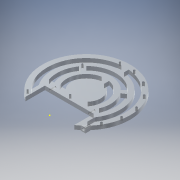
# Autodesk Inventor part: M02_R01 - Main Spherical Shaft
Saved by Autodesk Inventor 2016 (Build 200138000, 138)
## iProperties
Created: 2017-02-27
Part Number: M02_R01 - Main Spherical Shaft
Material: Glass
Document SubType Name: Modeling
Designer: Fernando
Stock Number: 0
Mass: 238.84 g
Surface Area: 460.743 cm^2
Volume: 109.56 cm^3
Density: 2.18 g/cm^3
Appearance: Clear
SurfaceArea_m2: .05
Author: Fernando
Autodesk Inventor part; units mm, degrees
ref_plane "YZ Plane" through (0, 0, 0) normal (1, 0, 0) x (0, 1, 0)
ref_plane "XZ Plane" through (0, 0, 0) normal (0, 1, 0) x (-1, 0, 0)
ref_plane "XY Plane" through (0, 0, 0) normal (0, 0, 1) x (1, 0, 0)
sketch "Sketch2" plane through (0, 0, 0) normal (0, 0, 1) x (1, 0, 0)
  line L0 (-50, 0) -> (50, 0) construction
  line L1 (50, 0) -> (50, 40)
  line L2 (50, 40) -> (-50, 40)
  line L3 (-50, 40) -> (-50, 0)
  arc A0 (50, 0) -> (-50, 0) centre (0, 74.8331) ccw
  line L4 (57.5, 19.2117) -> (57.5, 34.9113)
  line L5 (-57.5, 34.9113) -> (-57.5, 19.2117)
  line L6 (7.5, 154.4808) -> (7.5, 144.4302)
  line L7 (-7.5, 154.4808) -> (-7.5, 144.4302)
  line L8 (7.5, 144.4302) -> (-7.5, 154.4808) construction
  arc A1 (57.5, 34.9113) -> (7.5, 144.4302) centre (0, 74.8331) ccw
  arc A2 (-7.5, 144.4302) -> (-57.5, 34.9113) centre (0, 74.8331) ccw
  arc A3 (57.5, 19.2117) -> (7.5, 154.4808) centre (0, 74.8331) ccw
  arc A4 (-7.5, 154.4808) -> (-57.5, 19.2117) centre (0, 74.8331) ccw
  line L9 (56.6273, 55) -> (45.8982, 55)
  line L10 (-45.8982, 55) -> (-56.6273, 55)
  line L11 (42.4264, 117.2596) -> (35.3553, 110.1885)
  line L12 (-35.3553, 110.1885) -> (-42.4264, 117.2596)
  line L13 (49.1491, 109.2477) -> (40.9576, 103.512)
  line L14 (-49.1491, 109.2477) -> (-40.9576, 103.512)
  arc A5 (-40.9576, 103.512) -> (-45.8982, 55) centre (0, 74.8331) ccw
  arc A6 (-49.1491, 109.2477) -> (-56.6273, 55) centre (0, 74.8331) ccw
  arc A7 (45.8982, 55) -> (40.9576, 103.512) centre (0, 74.8331) ccw
  arc A8 (35.3553, 110.1885) -> (-35.3553, 110.1885) centre (0, 74.8331) ccw
  arc A9 (56.6273, 55) -> (49.1491, 109.2477) centre (0, 74.8331) ccw
  arc A10 (42.4264, 117.2596) -> (-42.4264, 117.2596) centre (0, 74.8331) ccw
  line L15 (7.5, 114.1237) -> (7.5, 103.8805)
  line L16 (-7.5, 103.8805) -> (-7.5, 114.1237)
  line L17 (34.7368, 55) -> (22.5088, 55)
  line L18 (-22.5088, 55) -> (-34.7368, 55)
  arc A11 (-7.5, 103.8805) -> (-22.5088, 55) centre (0, 74.8331) ccw
  arc A12 (22.5088, 55) -> (7.5, 103.8805) centre (0, 74.8331) ccw
  arc A13 (-7.5, 114.1237) -> (-34.7368, 55) centre (0, 74.8331) ccw
  arc A14 (34.7368, 55) -> (7.5, 114.1237) centre (0, 74.8331) ccw
  point P0 (0, 0)
  point P1 (0, 0)
  point P2 (0, 149.4555)
  dimension "d11" = 100
  dimension "d12" = 40
  dimension "d27" = 90
  dimension "d29" = 7.5
  dimension "d30" = 7.5
  dimension "d34" = 10
  dimension "d35" = 10
  dimension "d36" = 10
  dimension "d37" = 10
  dimension "d38" = 15
  dimension "d71" = 15
  dimension "d74" = 10
  dimension "d75" = 10
  dimension "d76" = 45
  dimension "d77" = 45
  dimension "d78" = 10
  dimension "d79" = 10
  dimension "d80" = 10
  dimension "d81" = 10
  constraints: 38 end point, 30 point on circle, 15 centre point, 7 coincident, 6 concentric, 5 collinear, 5 parallel, 4 point on line, 4 vertical, 3 horizontal, 2 midpoint, 1 perpendicular, 1 vertical alignment
  measures "d11" distance of L0.start L0.end
  measures "d12" distance of L0.end L1.end
  measures "d27" radius of A0
  measures "d29" distance between parallel lines of L1 L4
  measures "d30" distance between parallel lines of L3 L5
  measures "d34" radial gap between concentric circles of A0 A3
  measures "d35" radial gap between concentric circles of A3 A1
  measures "d36" radial gap between concentric circles of A4 A2
  measures "d37" radial gap between concentric circles of A0 A4
  measures "d38" distance between parallel lines of L7 L6
  measures "d71" distance between parallel lines of L2 L10
  measures "d74" angle of L13 L11
  measures "d75" angle of L14 L12
  measures "d76" angle of L2 L11
  measures "d77" angle of L2 L12
  measures "d78" radial gap between concentric circles of A1 A10
  measures "d79" radial gap between concentric circles of A8 A10
  measures "d80" radial gap between concentric circles of A7 A14
  measures "d81" radial gap between concentric circles of A12 A14
extrude "Extrusion2" add sketch "Sketch2" along normal mid plane 8
sketch "Sketch6" plane through (0, 0, 0) normal (0, 0, 1) x (1, 0, 0)
  arc A0 (50, 0) -> (-50, 0) centre (0, 74.8331) ccw projected
  line L0 (57.5, 5.5962) -> (67.5, 5.5962)
  line L1 (67.5, 5.5962) -> (67.5, 15.3037)
  point P0 (0, 0)
  point P1 (57.5, 19.2117)
  dimension "d48" = 10
  constraints: 4 end point, 2 point on circle, 1 horizontal, 1 perpendicular, 1 vertical alignment
  measures "d48" distance of L0.start L0.end
extrude "Extrusion4" add sketch "Sketch6" along normal mid plane 10
sketch "Sketch8" plane through (0, 0, 0) normal (0, 0, 1) x (1, 0, 0)
  arc A0 (50, 0) -> (-50, 0) centre (0, 74.8331) ccw construction
  line L0 (2, 165.8331) -> (0, 163.8331)
  line L1 (0, 163.8331) -> (-2, 165.8331)
  line L2 (-2, 165.8331) -> (2, 165.8331)
  line L3 (0, 165.8331) -> (0, 164.8331) construction
  point P0 (0, 0)
  point P1 (67.5, 15.3037)
  dimension "d67" = 1
  dimension "d68" = 2
  constraints: 8 end point, 2 perpendicular, 1 horizontal, 1 midpoint, 1 point on circle, 1 vertical, 1 vertical alignment
  measures "d67" distance of L3.start L3.end
  measures "d68" distance from line of L2 L0.end
extrude "Extrusion5" cut sketch "Sketch8" along normal mid plane 10
sketch "Sketch7" plane through (57.5, 5.5962, 5) normal (0, -1, 0) x (1, 0, 0)
  line L0 (10, 0) -> (10, -10) projected
  line L1 (0, 0) -> (10, 0) projected
  line L2 (10, -10) -> (0, -10) projected
  line L3 (0, 0) -> (10, -10)
  line L4 (0, -9) -> (0, -1) projected
  line L5 (0, -1) -> (0, 0) projected
  line L6 (0, -10) -> (0, -9) projected
  point P0 (-57.5, -5)
  point P1 (5, -5)
  constraints: 2 end point, 2 midpoint
hole "Hole2" at (62.5, 5.5962, 0) direction (0, 1, 0) diameter 5.5 depth 25 tip angle 118
sketch "Sketch9" plane through (0, 0, -4) normal (0, 0, -1) x (-1, 0, 0)
  arc A0 (-0.9945, 164.8277) -> (-67.5, 15.3037) centre (0, 74.8331) ccw construction
  line L0 (-73.6122, 32.3331) -> (0, 74.8331) construction
  line L1 (0, 74.8331) -> (0, 98.0248) construction
  point P0 (0, 0)
  dimension "d82" = 85
  dimension "d83" = 120
  constraints: 4 end point, 1 vertical
  measures "d82" distance of L0.start L0.end
  measures "d83" angle of L0 L1
hole "Hole3" at (73.6122, 32.3331, -4) direction (0, 0, 1) diameter 4.5 depth 10 tip angle 118
pattern_circular "Circular Pattern2" count 6 over 110 about axis through (0, 74.8331, 0) along (0, 0, 1) of "Hole3"
sketch "Sketch10" plane through (-50, 40, 4) normal (0, -1, 0) x (1, 0, 0)
  line L0 (90, -4.6611) -> (50, -4) construction
  line L1 (50, -4) -> (10, -3.3389) construction
  dimension "d94" = 80
  constraints: 4 end point, 2 collinear
  measures "d94" horizontal distance of L0.start L1.end
hole "Hole4" at (-40, 40, 0.6611) at (40, 40, -0.6611) direction (0, 1, 0) diameter 3.242 depth 11.8 tip angle 118 thread size "M4x0.7" class "6H" standard "ISO Metric profile"
sketch "Sketch11" plane through (0, 0, -4) normal (0, 0, -1) x (-1, 0, 0)
  point P0 (0, 0)
sketch "Sketch12" plane through (0, 0, -4) normal (0, 0, -1) x (-1, 0, 0)
  arc A0 (22.5088, 55) -> (7.5, 103.8805) centre (0, 74.8331) ccw construction
  line L0 (0, 74.8331) -> (12.608, 74.8331) construction
  point P0 (0, 0)
  point P1 (14.7601, 158.5418)
  point P2 (60.1041, 14.7291)
  point P3 (49.7929, 116.6143)
  point P4 (8, 49.8331)
  dimension "d102" = 85
  dimension "d103" = 65
  dimension "d104" = 85
  dimension "d105" = 80
  dimension "d106" = 40
  dimension "d107" = 45
  dimension "d108" = 25
  dimension "d109" = 8
  constraints: 2 end point, 1 horizontal
  measures "d102" distance of L0.start point (14.76, 158.542)
  measures "d103" distance of L0.start point (49.793, 116.614)
  measures "d104" distance of point (60.104, 14.729) L0.start
  measures "d108" distance from line of point (8, 49.833) L0
  measures "d109" horizontal distance of L0.start point (8, 49.833)
hole "Hole5" at (-14.7601, 158.5418, -4) at (-49.7929, 116.6143, -4) at (-8, 49.8331, -4) at (-60.1041, 14.7291, -4) direction (0, 0, 1) diameter 3.5 depth 11.8 tip angle 118
equation "\"d36\" = d35"
equation "\"d37\" = d34"
body "Solid2"
